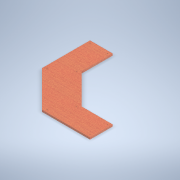
# Autodesk Inventor part: Tapa02
Saved by Autodesk Inventor 2020.3 (Build 243373000, 373)
## iProperties
Created: 2020-11-12
Part Number: Tapa02
Material: Madera (roble)
Document SubType Name: Modeling
Designer: codig
Density: 0.76 g/cm^3
Appearance: Roble blanco - Natural brillo medio
Author: codig
Autodesk Inventor part; units mm, degrees
ref_plane "YZ Plane" through (0, 0, 0) normal (1, 0, 0) x (0, 1, 0)
ref_plane "XZ Plane" through (0, 0, 0) normal (0, 1, 0) x (-1, 0, 0)
ref_plane "XY Plane" through (0, 0, 0) normal (0, 0, 1) x (1, 0, 0)
sketch "Boceto1" plane through (0, 0, 0) normal (0, 1, 0) x (-1, 0, 0)
  line L0 (-183.5, 200) -> (-183.5, 420)
  line L1 (-183.5, 420) -> (-483.5, 420)
  line L2 (-1000, 1016.5) -> (-780, 1016.5)
  line L3 (-1000, 1016.5) -> (-780, 1016.5) construction
  line L4 (-780, 1016.5) -> (-780, 716.5)
  line L5 (-780, 716.5) -> (-483.5, 420)
  line L6 (-1000, 1016.5) -> (-1000, 550)
  line L7 (-183.5, 200) -> (-650, 200)
  line L8 (-650, 200) -> (-1000, 550)
  line L9 (-1000, 1016.5) -> (-964.644, 1016.5) construction
  circle A0 centre (-974.9995, 991.4995) radius 4
  circle A1 centre (-805.0005, 991.4995) radius 4
  circle A2 centre (-974.9995, 575.0005) radius 4
  circle A3 centre (-805.0005, 691.4995) radius 4
  circle A4 centre (-508.5005, 394.9995) radius 4
  circle A5 centre (-624.9995, 225.0005) radius 4
  circle A6 centre (-208.5005, 225.0005) radius 4
  circle A7 centre (-208.5005, 394.9995) radius 4
  constraints: 20 end point, 8 centre point, 4 horizontal, 2 perpendicular, 1 collinear
extrude "Extrusión2" add sketch "Boceto1" along normal blind 18
